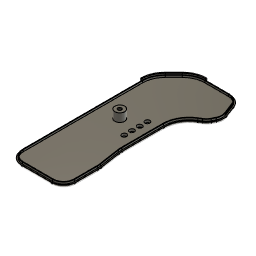
thumbwheelTop v11 (Autodesk Fusion 360 design; units mm, degrees)
Autodesk Fusion 360 part; units mm, degrees
sketch "Sketch1" plane through (0, 0, 0) normal (0, 1, 0) x (1, 0, 0)
  line L0 (31.7101, -12.3063) -> (34.0314, -10.9136)
  arc A0 (39.2196, -4.033) -> (39.6234, 3.9906) centre (30.2753, 0.4391) ccw
  line L1 (37.8307, -6.8108) -> (39.2196, -4.033)
  arc A1 (15, -115) -> (25, -105) centre (15, -105) ccw
  arc A2 (31.7101, -12.3063) -> (22, -29.4562) centre (42, -29.4562) ccw
  arc A3 (34.0314, -10.9136) -> (37.8307, -6.8108) centre (28.8864, -2.3386) ccw
  arc A4 (36.181, 13.0515) -> (26.8329, 19.5) centre (26.8329, 9.5) ccw
  line L2 (39.6234, 3.9906) -> (36.181, 13.0515)
  arc A5 (-13.6421, 6.6863) -> (-19.5, -7.4558) centre (0.5, -7.4558) ccw
  line L3 (22, -63.3592) -> (22, -29.4562)
  arc A6 (7.4558, 19.5) -> (-6.6863, 13.6421) centre (7.4558, -0.5) ccw
  line L4 (24.7787, -83.3757) -> (22.2213, -66.326)
  arc A7 (25, -86.3425) -> (24.7787, -83.3757) centre (5, -86.3425) ccw
  line L5 (-6.6863, 13.6421) -> (-13.6421, 6.6863)
  line L6 (-9.5, -115) -> (15, -115)
  arc A8 (-19.5, -105) -> (-9.5, -115) centre (-9.5, -105) ccw
  line L7 (25, -105) -> (25, -86.3425)
  line L8 (26.8329, 19.5) -> (7.4558, 19.5)
  line L9 (-19.5, -7.4558) -> (-19.5, -105)
  arc A9 (22, -63.3592) -> (22.2213, -66.326) centre (42, -63.3592) ccw
extrude "Extrude1" add sketch "Sketch1" along normal blind 2
sketch "Sketch2" plane through (0, 2, 0) normal (0, 1, 0) x (-1, 0, 0)
  line L0 (-31.7101, 12.3063) -> (-34.0314, 10.9136)
  arc A0 (-34.0314, 10.9136) -> (-37.8307, 6.8108) centre (-28.8864, 2.3386) ccw
  line L1 (-37.8307, 6.8108) -> (-39.2196, 4.033)
  arc A1 (-39.2196, 4.033) -> (-39.6234, -3.9906) centre (-30.2753, -0.4391) ccw
  line L2 (-39.6234, -3.9906) -> (-36.181, -13.0515)
  arc A2 (-36.181, -13.0515) -> (-26.8329, -19.5) centre (-26.8329, -9.5) ccw
  line L3 (-26.8329, -19.5) -> (-7.4558, -19.5)
  arc A3 (-7.4558, -19.5) -> (6.6863, -13.6421) centre (-7.4558, 0.5) ccw
  line L4 (6.6863, -13.6421) -> (13.6421, -6.6863)
  arc A4 (13.6421, -6.6863) -> (19.5, 7.4558) centre (-0.5, 7.4558) ccw
  line L5 (19.5, 7.4558) -> (19.5, 105)
  arc A5 (19.5, 105) -> (9.5, 115) centre (9.5, 105) ccw
  line L6 (9.5, 115) -> (-15, 115)
  arc A6 (-15, 115) -> (-25, 105) centre (-15, 105) ccw
  line L7 (-25, 105) -> (-25, 86.3425)
  arc A7 (-25, 86.3425) -> (-24.7787, 83.3757) centre (-5, 86.3425) ccw
  line L8 (-24.7787, 83.3757) -> (-22.2213, 66.326)
  arc A8 (-22, 63.3592) -> (-22.2213, 66.326) centre (-42, 63.3592) ccw
  line L9 (-22, 63.3592) -> (-22, 29.4562)
  arc A9 (-31.7101, 12.3063) -> (-22, 29.4562) centre (-42, 29.4562) ccw
  line L10 (18.5, 7.4558) -> (18.5, 105)
  arc A10 (18.5, 105) -> (9.5, 114) centre (9.5, 105) ccw
  line L11 (9.5, 114) -> (-15, 114)
  arc A11 (-15, 114) -> (-24, 105) centre (-15, 105) ccw
  line L12 (-24, 105) -> (-24, 86.3425)
  arc A12 (-24, 86.3425) -> (-23.7898, 83.524) centre (-5, 86.3425) ccw
  line L13 (-23.7898, 83.524) -> (-21.2323, 66.4743)
  arc A13 (-21, 63.3592) -> (-21.2323, 66.4743) centre (-42, 63.3592) ccw
  line L14 (-21, 63.3592) -> (-21, 29.4562)
  arc A14 (-31.1956, 11.4488) -> (-21, 29.4562) centre (-42, 29.4562) ccw
  line L15 (-31.1956, 11.4488) -> (-33.5169, 10.0561)
  arc A15 (-33.5169, 10.0561) -> (-36.9363, 6.3636) centre (-28.8864, 2.3386) ccw
  line L16 (-36.9363, 6.3636) -> (-38.3251, 3.5858)
  arc A16 (-38.3251, 3.5858) -> (-38.6886, -3.6354) centre (-30.2753, -0.4391) ccw
  line L17 (-38.6886, -3.6354) -> (-35.2462, -12.6963)
  arc A17 (-35.2462, -12.6963) -> (-26.8329, -18.5) centre (-26.8329, -9.5) ccw
  line L18 (-26.8329, -18.5) -> (-7.4558, -18.5)
  arc A18 (-7.4558, -18.5) -> (5.9792, -12.935) centre (-7.4558, 0.5) ccw
  line L19 (5.9792, -12.935) -> (12.935, -5.9792)
  arc A19 (12.935, -5.9792) -> (18.5, 7.4558) centre (-0.5, 7.4558) ccw
  line L20 (9.5, 113.5) -> (-15, 113.5)
  arc A20 (-15, 113.5) -> (-23.5, 105) centre (-15, 105) ccw
  line L21 (-23.5, 105) -> (-23.5, 86.3425)
  arc A21 (-23.5, 86.3425) -> (-23.2953, 83.5982) centre (-5, 86.3425) ccw
  line L22 (-23.2953, 83.5982) -> (-20.7379, 66.5485)
  arc A22 (-20.5, 63.3592) -> (-20.7379, 66.5485) centre (-42, 63.3592) ccw
  line L23 (-20.5, 63.3592) -> (-20.5, 29.4562)
  arc A23 (-30.9383, 11.0201) -> (-20.5, 29.4562) centre (-42, 29.4562) ccw
  line L24 (-30.9383, 11.0201) -> (-33.2596, 9.6273)
  arc A24 (-33.2596, 9.6273) -> (-36.489, 6.1399) centre (-28.8864, 2.3386) ccw
  line L25 (-36.489, 6.1399) -> (-37.8779, 3.3622)
  arc A25 (-37.8779, 3.3622) -> (-38.2212, -3.4579) centre (-30.2753, -0.4391) ccw
  line L26 (-38.2212, -3.4579) -> (-34.7788, -12.5188)
  arc A26 (-34.7788, -12.5188) -> (-26.8329, -18) centre (-26.8329, -9.5) ccw
  line L27 (-26.8329, -18) -> (-7.4558, -18)
  arc A27 (-7.4558, -18) -> (5.6256, -12.5815) centre (-7.4558, 0.5) ccw
  line L28 (5.6256, -12.5815) -> (12.5815, -5.6256)
  arc A28 (12.5815, -5.6256) -> (18, 7.4558) centre (-0.5, 7.4558) ccw
  line L29 (18, 7.4558) -> (18, 105)
  arc A29 (18, 105) -> (9.5, 113.5) centre (9.5, 105) ccw
  dimension "d40" = -1
  dimension "d41" = -1.5
extrude "Extrude2" add sketch "Sketch2" along normal blind 1.5 contours L10 A10 L11 A11 L12 A12 L13 A13 L14 A14 L15 A15 L16 A16 L17 A17 L18 A18 L19 A19
sketch "Sketch3" plane through (0, 2, 0) normal (0, 1, 0) x (-1, 0, 0)
  line L0 (19.5, 7.4558) -> (18.5, 7.4558)
  arc A0 (-31.7101, 12.3063) -> (-22, 29.4562) centre (-42, 29.4562) ccw
  line L1 (-31.7101, 12.3063) -> (-34.0314, 10.9136)
  arc A1 (-34.0314, 10.9136) -> (-37.8307, 6.8108) centre (-28.8864, 2.3386) ccw
  line L2 (-37.8307, 6.8108) -> (-39.2196, 4.033)
  line L3 (-25, 105) -> (-25, 86.3425)
  arc A2 (-25, 86.3425) -> (-24.7787, 83.3757) centre (-5, 86.3425) ccw
  line L4 (-24.7787, 83.3757) -> (-22.2213, 66.326)
  arc A3 (-22, 63.3592) -> (-22.2213, 66.326) centre (-42, 63.3592) ccw
  line L5 (-22, 63.3592) -> (-22, 29.4562)
  line L6 (-39.6234, -3.9906) -> (-36.181, -13.0515)
  arc A4 (-36.181, -13.0515) -> (-26.8329, -19.5) centre (-26.8329, -9.5) ccw
  line L7 (-26.8329, -19.5) -> (-7.4558, -19.5)
  arc A5 (-7.4558, -19.5) -> (6.6863, -13.6421) centre (-7.4558, 0.5) ccw
  line L8 (6.6863, -13.6421) -> (13.6421, -6.6863)
  arc A6 (13.6421, -6.6863) -> (19.5, 7.4558) centre (-0.5, 7.4558) ccw
  line L9 (19.5, 7.4558) -> (19.5, 105)
  arc A7 (19.5, 105) -> (9.5, 115) centre (9.5, 105) ccw
  line L10 (9.5, 115) -> (-15, 115)
  arc A8 (-15, 115) -> (-25, 105) centre (-15, 105) ccw
  arc A9 (-33.2596, 9.6273) -> (-36.489, 6.1399) centre (-28.8864, 2.3386) ccw
  line L11 (-36.489, 6.1399) -> (-37.8779, 3.3622)
  arc A10 (-37.8779, 3.3622) -> (-38.2212, -3.4579) centre (-30.2753, -0.4391) ccw
  line L12 (-38.2212, -3.4579) -> (-34.7788, -12.5188)
  arc A11 (-34.7788, -12.5188) -> (-26.8329, -18) centre (-26.8329, -9.5) ccw
  line L13 (-26.8329, -18) -> (-7.4558, -18)
  arc A12 (-7.4558, -18) -> (5.6256, -12.5815) centre (-7.4558, 0.5) ccw
  line L14 (5.6256, -12.5815) -> (12.5815, -5.6256)
  arc A13 (12.5815, -5.6256) -> (18, 7.4558) centre (-0.5, 7.4558) ccw
  line L15 (18, 7.4558) -> (18, 105)
  arc A14 (18, 105) -> (9.5, 113.5) centre (9.5, 105) ccw
  line L16 (9.5, 113.5) -> (-15, 113.5)
  arc A15 (-15, 113.5) -> (-23.5, 105) centre (-15, 105) ccw
  line L17 (-23.5, 105) -> (-23.5, 86.3425)
  arc A16 (-23.5, 86.3425) -> (-23.2953, 83.5982) centre (-5, 86.3425) ccw
  line L18 (-23.2953, 83.5982) -> (-20.7379, 66.5485)
  arc A17 (-20.5, 63.3592) -> (-20.7379, 66.5485) centre (-42, 63.3592) ccw
  line L19 (-20.5, 63.3592) -> (-20.5, 29.4562)
  arc A18 (-30.9383, 11.0201) -> (-20.5, 29.4562) centre (-42, 29.4562) ccw
  line L20 (-30.9383, 11.0201) -> (-33.2596, 9.6273)
  arc A19 (-39.2196, 4.033) -> (-39.6234, -3.9906) centre (-30.2753, -0.4391) ccw
  arc A20 (-31.1956, 11.4488) -> (-21, 29.4562) centre (-42, 29.4562) ccw
  line L21 (-21, 29.4562) -> (-21, 63.3592)
  arc A21 (-21, 63.3592) -> (-21.2323, 66.4743) centre (-42, 63.3592) ccw
  line L22 (-21.2323, 66.4743) -> (-23.7898, 83.524)
  arc A22 (-24, 86.3425) -> (-23.7898, 83.524) centre (-5, 86.3425) ccw
  line L23 (-24, 86.3425) -> (-24, 105)
  arc A23 (-15, 114) -> (-24, 105) centre (-15, 105) ccw
  line L24 (-15, 114) -> (9.5, 114)
  arc A24 (18.5, 105) -> (9.5, 114) centre (9.5, 105) ccw
  line L25 (18.5, 105) -> (18.5, 7.4558)
  arc A25 (12.935, -5.9792) -> (18.5, 7.4558) centre (-0.5, 7.4558) ccw
  line L26 (12.935, -5.9792) -> (5.9792, -12.935)
  arc A26 (-7.4558, -18.5) -> (5.9792, -12.935) centre (-7.4558, 0.5) ccw
  line L27 (-7.4558, -18.5) -> (-26.8329, -18.5)
  arc A27 (-35.2462, -12.6963) -> (-26.8329, -18.5) centre (-26.8329, -9.5) ccw
  line L28 (-35.2462, -12.6963) -> (-38.6886, -3.6354)
  arc A28 (-38.3251, 3.5858) -> (-38.6886, -3.6354) centre (-30.2753, -0.4391) ccw
  line L29 (-38.3251, 3.5858) -> (-36.9363, 6.3636)
  arc A29 (-33.5169, 10.0561) -> (-36.9363, 6.3636) centre (-28.8864, 2.3386) ccw
  line L30 (-33.5169, 10.0561) -> (-31.1956, 11.4488)
  line L31 (-7.4558, -18.5) -> (-7.4558, -19.5)
  constraint coincident A26.start L27.start
  constraint coincident L7.end A5.start
extrude "Extrude3" add sketch "Sketch3" along normal blind 2.6 contours L0 A5 L8 A6 A25 L26 A26 L31
sketch "Sketch4" plane through (0, 0, 0) normal (0, -1, 0) x (1, 0, 0)
  circle A0 centre (11.5, 33) radius 2
  circle A1 centre (11.5, 39.3) radius 2
  circle A2 centre (11.5, 45.6) radius 2
  circle A3 centre (11.5, 51.9) radius 2
  line L0 (34.0314, 10.9136) -> (31.7101, 12.3063)
  arc A4 (22, 29.4562) -> (31.7101, 12.3063) centre (42, 29.4562) ccw
  line L1 (22, 29.4562) -> (22, 63.3592)
  arc A5 (22.2213, 66.326) -> (22, 63.3592) centre (42, 63.3592) ccw
  line L2 (22.2213, 66.326) -> (24.7787, 83.3757)
  arc A6 (24.7787, 83.3757) -> (25, 86.3425) centre (5, 86.3425) ccw
  line L3 (25, 86.3425) -> (25, 105)
  arc A7 (25, 105) -> (15, 115) centre (15, 105) ccw
  line L4 (15, 115) -> (-9.5, 115)
  arc A8 (-9.5, 115) -> (-19.5, 105) centre (-9.5, 105) ccw
  line L5 (-19.5, 105) -> (-19.5, 7.4558)
  arc A9 (-19.5, 7.4558) -> (-13.6421, -6.6863) centre (0.5, 7.4558) ccw
  line L6 (-13.6421, -6.6863) -> (-6.6863, -13.6421)
  arc A10 (-6.6863, -13.6421) -> (7.4558, -19.5) centre (7.4558, 0.5) ccw
  line L7 (7.4558, -19.5) -> (26.8329, -19.5)
  arc A11 (26.8329, -19.5) -> (36.181, -13.0515) centre (26.8329, -9.5) ccw
  line L8 (36.181, -13.0515) -> (39.6234, -3.9906)
  arc A12 (39.6234, -3.9906) -> (39.2196, 4.033) centre (30.2753, -0.4391) ccw
  line L9 (39.2196, 4.033) -> (37.8307, 6.8108)
  arc A13 (37.8307, 6.8108) -> (34.0314, 10.9136) centre (28.8864, 2.3386) ccw
  dimension "d14" = 4
  dimension "d18" = 0
  dimension "d19" = 6.3
  dimension "d44" = 10.5
  measures "d14" diameter of A0
  measures "d44" distance of A0.centre L1
extrude "Extrude4" cut sketch "Sketch4" against normal blind 5 contours A0 | A1 | A2 | A3
sketch "Sketch5" plane through (0, 2, 0) normal (0, 1, 0) x (-1, 0, 0)
  circle A0 centre (-11.5, 39.3) radius 2
  circle A1 centre (-11.5, 45.6) radius 2
  circle A2 centre (-11.5, 33) radius 2
  circle A3 centre (-11.5, 51.9) radius 2
  circle A4 centre (2.08, 42.036) radius 3
  circle A5 centre (2.08, 42.036) radius 4
  arc A6 (-33.2596, 9.6273) -> (-36.489, 6.1399) centre (-28.8864, 2.3386) ccw
  line L0 (-36.489, 6.1399) -> (-37.8779, 3.3622)
  arc A7 (-37.8779, 3.3622) -> (-38.2212, -3.4579) centre (-30.2753, -0.4391) ccw
  line L1 (-38.2212, -3.4579) -> (-34.7788, -12.5188)
  arc A8 (-34.7788, -12.5188) -> (-26.8329, -18) centre (-26.8329, -9.5) ccw
  line L2 (-26.8329, -18) -> (-7.4558, -18)
  arc A9 (-7.4558, -18) -> (5.6256, -12.5815) centre (-7.4558, 0.5) ccw
  line L3 (5.6256, -12.5815) -> (12.5815, -5.6256)
  arc A10 (12.5815, -5.6256) -> (18, 7.4558) centre (-0.5, 7.4558) ccw
  line L4 (18, 7.4558) -> (18, 105)
  arc A11 (18, 105) -> (9.5, 113.5) centre (9.5, 105) ccw
  arc A12 (-15, 113.5) -> (-23.5, 105) centre (-15, 105) ccw
  line L5 (-23.5, 105) -> (-23.5, 86.3425)
  arc A13 (-23.5, 86.3425) -> (-23.2953, 83.5982) centre (-5, 86.3425) ccw
  line L6 (-23.2953, 83.5982) -> (-20.7379, 66.5485)
  arc A14 (-20.5, 63.3592) -> (-20.7379, 66.5485) centre (-42, 63.3592) ccw
  line L7 (-20.5, 63.3592) -> (-20.5, 29.4562)
  arc A15 (-30.9383, 11.0201) -> (-20.5, 29.4562) centre (-42, 29.4562) ccw
  line L8 (-30.9383, 11.0201) -> (-33.2596, 9.6273)
  line L9 (19.5, 7.4558) -> (19.5, 105)
  line L10 (9.5, 115) -> (-15, 115)
  dimension "d22" = 6
  dimension "d23" = 8
  dimension "d42" = 17.42
  dimension "d43" = 72.964
  constraint concentric A4 A5
  measures "d22" diameter of A4
  measures "d23" diameter of A5
  measures "d42" distance of A4.centre L9
  measures "d43" distance of A4.centre L10
extrude "Extrude5" add sketch "Sketch5" along normal blind 6.8 contours A5
extrude "Extrude6" cut 1 faces at (-1.2923, 2, 40.6272) along direction (0, -1, 0) blind 5
sketch "Sketch6" plane through (0, 8.8, 0) normal (0, 1, 0) x (-1, 0, 0)
  circle A0 centre (2.08, 42.036) radius 3
  circle A1 centre (2.08, 42.036) radius 4
  circle A2 centre (2.08, 42.036) radius 4
extrude "Extrude7" add sketch "Sketch6" against normal blind 1 contours A0 | A1 A2
sketch "Sketch7" plane through (0, 8.8, 0) normal (0, 1, 0) x (-1, 0, 0)
  circle A0 centre (2.08, 42.036) radius 4
  circle A1 centre (2.08, 42.036) radius 1.5
  dimension "d31" = 3
  constraint concentric A0 A1
  measures "d31" diameter of A1
extrude "Extrude8" cut sketch "Sketch7" against normal blind 5 contours A1
fillet "Fillet1" radius 2 20 edges at (23.5, 0, 74.8508) (22.0554, 0, 64.8467) (22, 0, 46.4077) (24.596, 0, 19.6022) (32.8707, 0, 11.6099) (36.2236, 0, 9.1331) (38.5251, 0, 5.4219) (40.2626, 0, 0.0635) (37.9022, 0, -8.521) (32.5112, 0, -17.7315) (17.1444, 0, -19.5) (-0.1978, 0, -17.9776) (-10.1642, 0, -10.1642) (-17.9776, 0, -0.1978) (-19.5, 0, 56.2279) (-16.5711, 0, 112.0711) (2.75, 0, 115) (22.0711, 0, 112.0711) (25, 0, 95.6712) (24.9446, 0, 84.855)
